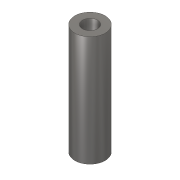
# Autodesk Inventor part: Rändelgriff
Saved by Autodesk Inventor 2018.3 (Build 223284000, 284)
## iProperties
Created: 2019-11-28
Material: Stahl, Legierung
Document SubType Name: Modeling
Designer: dirkb
Density: 7.73 g/cm^3
Appearance: Halbpoliert
Description: Rändelgriff
Werkstoff: X8CrNiS18-9
Author: dirkb
Autodesk Inventor part; units mm, degrees
ref_plane "YZ Plane" through (0, 0, 0) normal (1, 0, 0) x (0, 1, 0)
ref_plane "XZ Plane" through (0, 0, 0) normal (0, 1, 0) x (-1, 0, 0)
ref_plane "XY Plane" through (0, 0, 0) normal (0, 0, 1) x (1, 0, 0)
sketch "Skizze_Grudnkörper" plane through (0, 0, 0) normal (0, 0, 1) x (1, 0, 0)
  circle A0 centre (0, 0) radius 4
  dimension "d0" = 8
  constraints: 1 centre point, 1 coincident
  measures "d0" diameter of A0
extrude "Grundkörper" add sketch "Skizze_Grudnkörper" along normal blind 30
hole "Bohrung_4_mm" at (0, 0, 30) direction (0, 0, -1) diameter 4 depth 10 tip angle 118
sketch "Skizze2" plane through (0, 0, 0) normal (0, 1, 0) x (-1, 0, 0)
  line L0 (-4, 0) -> (-4, 30) projected
  line L1 (-4, 30) -> (-2, 30) projected
  line L2 (-2, 30) -> (-2, 20) projected
  line L3 (-2, 20) -> (0, 18.7983) projected
  line L4 (0, 18.7983) -> (2, 20) projected
  line L5 (2, 20) -> (2, 30) projected
  line L6 (2, 30) -> (4, 30) projected
  line L7 (4, 30) -> (4, 0) projected
  line L8 (4, 0) -> (-4, 0) projected
  line L9 (5.6, 0) -> (-5.6, 0) projected
  line L10 (0, -6) -> (0, 36) projected
  circle A0 centre (0, 10) radius 10
  point P0 (0, 0)
  point P1 (4, 0.8348)
  point P2 (0, 0)
  dimension "d12" = 20
  constraints: 2 coincident, 2 point on circle, 2 point on line, 1 centre point
  measures "d12" diameter of A0
revolve "Kugel" cut sketch "Skizze2" angle 360 about axis through (0, 0, -10) along (0, 0, 1) contours A0 L7 L8
